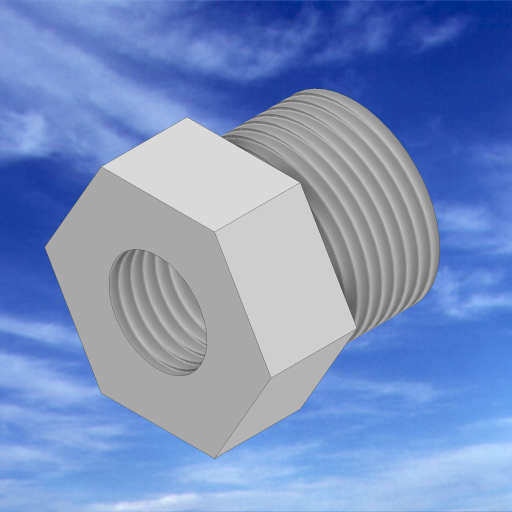
# Autodesk Inventor part: HUDSON-1-47
Saved by Autodesk Inventor 2024.2 (Build 282272000, 272)
## iProperties
Created: 2024-10-10
Part Number: HUDSON-1-47
Material: Generic
Document SubType Name: Modeling
Designer: Precisión-05
Density: 1 g/cm^3
Appearance: Default
Author: Precisión-05
Autodesk Inventor part; units mm, degrees
ref_plane "YZ Plane" through (0, 0, 0) normal (1, 0, 0) x (0, 1, 0)
ref_plane "XZ Plane" through (0, 0, 0) normal (0, 1, 0) x (-1, 0, 0)
ref_plane "XY Plane" through (0, 0, 0) normal (0, 0, 1) x (1, 0, 0)
sketch "Sketch1" plane through (0, 0, 0) normal (0, 1, 0) x (-1, 0, 0)
  line L0 (9.2376, 0) -> (4.6188, -8)
  line L1 (4.6188, -8) -> (-4.6188, -8)
  line L2 (-4.6188, -8) -> (-9.2376, 0)
  line L3 (-9.2376, 0) -> (-4.6188, 8)
  line L4 (-4.6188, 8) -> (4.6188, 8)
  line L5 (4.6188, 8) -> (9.2376, 0)
  point P0 (0, 0)
  point P1 (0, 0)
  dimension "d0" = 16
  constraints: 12 end point, 1 coincident, 13 other
  measures "d0" distance of L0.end L4.end
extrude "Extrusion1" add sketch "Sketch1" along normal blind 7
sketch "Sketch2" plane through (0, 7, 0) normal (0, 1, 0) x (1, 0, 0)
  circle A0 centre (0, 0) radius 7
  circle A1 centre (0, 0) radius 3.5
  dimension "d3" = 14
  dimension "d4" = 7
  constraints: 2 centre point, 2 coincident
  measures "d3" diameter of A0
  measures "d4" diameter of A1
extrude "Extrusion2" add sketch "Sketch2" along normal blind 9
thread "Thread1" size "M14x1" class "6g" standard "ANSI Metric M Profile" length 45
sketch "Sketch3" plane through (0, 16, 0) normal (0, 1, 0) x (1, 0, 0)
  circle A0 centre (0, 0) radius 5
  dimension "d9" = 10
  constraints: 1 centre point, 1 coincident
  measures "d9" diameter of A0
extrude "Extrusion3" cut sketch "Sketch3" against normal blind 6
sketch "Sketch4" plane through (0, 0, 0) normal (0, -1, 0) x (1, 0, 0)
  circle A0 centre (0, 0) radius 4
  dimension "d12" = 8
  constraints: 1 centre point, 1 coincident
  measures "d12" diameter of A0
extrude "Extrusion4" cut sketch "Sketch4" against normal blind 7
thread "Thread2" size "M8x1" class "6H" standard "ANSI Metric M Profile" length 45
body "Solid1"
